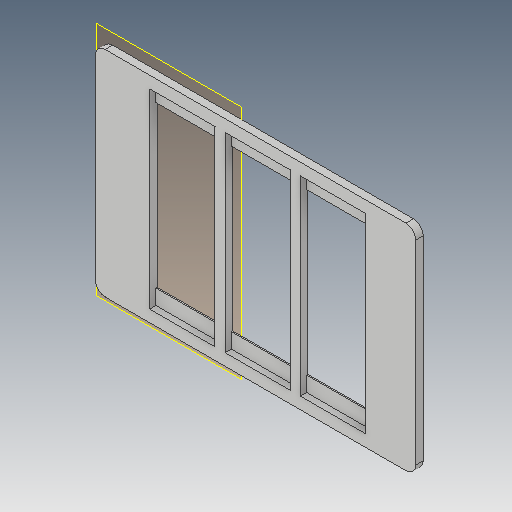
# Autodesk Inventor part: 30_MTP_wellplate_to_sample_adapter
Saved by Autodesk Inventor 2019.4 (Build 234330000, 330)
## iProperties
Created: 2021-05-14
Part Number: 30_MTP_wellplate_to_sample_adapter
Material: Generic
Document SubType Name: Modeling
Designer: diederichbenedict
Density: 1 g/cm^3
Appearance: Default
Author: diederichbenedict
Autodesk Inventor part; units mm, degrees
(part 1 of 2)
ref_plane "YZ Plane" through (0, 0, 0) normal (1, 0, 0) x (0, 1, 0)
ref_plane "XZ Plane" through (0, 0, 0) normal (0, 1, 0) x (-1, 0, 0)
ref_plane "XY Plane" through (0, 0, 0) normal (0, 0, 1) x (1, 0, 0)
ref_plane "Work Plane1" through (-0.8521, 0, -25.0767) normal (0, 0, 1) x (1, 0, 0)
sketch "Sketch1" plane through (-0.8521, 0, -25.0767) normal (0, 0, 1) x (1, 0, 0)
  line L0 (-59.9, 42.7) -> (-11.2, 42.7) projected
  arc A0 (-59.9, 42.7) -> (-63.8, 38.8) centre (-59.9, 38.8) ccw projected
  line L1 (-63.8, -38.8) -> (-63.8, 38.8) projected
  arc A1 (-63.8, -38.8) -> (-59.9, -42.7) centre (-59.9, -38.8) ccw projected
  line L2 (-11.2, -42.7) -> (-59.9, -42.7) projected
  line L3 (-11.2, -41.2) -> (-11.2, -42.7) projected
  line L4 (-55.7858, -41.2) -> (-11.2, -41.2) projected
  arc A2 (-56.5636, -40.8778) -> (-55.7858, -41.2) centre (-55.7858, -40.1) ccw projected
  line L5 (-61.9778, -35.4636) -> (-56.5636, -40.8778) projected
  arc A3 (-62.3, -34.6858) -> (-61.9778, -35.4636) centre (-61.2, -34.6858) ccw projected
  line L6 (-62.3, 34.6858) -> (-62.3, -34.6858) projected
  arc A4 (-61.9778, 35.4636) -> (-62.3, 34.6858) centre (-61.2, 34.6858) ccw projected
  line L7 (-56.5636, 40.8778) -> (-61.9778, 35.4636) projected
  arc A5 (-55.7858, 41.2) -> (-56.5636, 40.8778) centre (-55.7858, 40.1) ccw projected
  line L8 (-11.2, 41.2) -> (-55.7858, 41.2) projected
  line L9 (-11.2, 42.7) -> (-11.2, 41.2) projected
  line L10 (11.2, 42.7) -> (59.9, 42.7) projected
  line L11 (11.2, 41.2) -> (11.2, 42.7) projected
  line L12 (60.2, 41.2) -> (11.2, 41.2) projected
  arc A6 (62.3, 39.1) -> (60.2, 41.2) centre (60.2, 39.1) ccw projected
  line L13 (62.3, -39.1) -> (62.3, 39.1) projected
  arc A7 (60.2, -41.2) -> (62.3, -39.1) centre (60.2, -39.1) ccw projected
  line L14 (11.2, -41.2) -> (60.2, -41.2) projected
  line L15 (11.2, -42.7) -> (11.2, -41.2) projected
  line L16 (59.9, -42.7) -> (11.2, -42.7) projected
  arc A8 (59.9, -42.7) -> (63.8, -38.8) centre (59.9, -38.8) ccw projected
  line L17 (63.8, 38.8) -> (63.8, -38.8) projected
  arc A9 (63.8, 38.8) -> (59.9, 42.7) centre (59.9, 38.8) ccw projected
  line L18 (-11.2, 42.7) -> (11.2, 42.7)
  line L19 (-11.2, -42.7) -> (11.2, -42.7)
  point P0 (0.8521, 0)
  constraints: 4 end point, 1 horizontal, 1 parallel
extrude "Extrusion1" add sketch "Sketch1" along normal blind 3
sketch "Sketch2" plane through (-0.8521, 0, -22.0767) normal (0, 0, 1) x (1, 0, 0)
  line L0 (-61.4, -34.7272) -> (-61.4, 34.7272)
  arc A0 (-61.4, -34.7272) -> (-61.3707, -34.7979) centre (-61.3, -34.7272) ccw
  line L1 (-55.8979, -40.2707) -> (-61.3707, -34.7979)
  arc A1 (-55.8979, -40.2707) -> (-55.8272, -40.3) centre (-55.8272, -40.2) ccw
  line L2 (60.2, -40.3) -> (-55.8272, -40.3)
  arc A2 (60.2, -40.3) -> (61.4, -39.1) centre (60.2, -39.1) ccw
  line L3 (61.4, 39.1) -> (61.4, -39.1)
  arc A3 (61.4, 39.1) -> (60.2, 40.3) centre (60.2, 39.1) ccw
  line L4 (-55.8272, 40.3) -> (60.2, 40.3)
  arc A4 (-55.8272, 40.3) -> (-55.8979, 40.2707) centre (-55.8272, 40.2) ccw
  line L5 (-61.3707, 34.7979) -> (-55.8979, 40.2707)
  arc A5 (-61.3707, 34.7979) -> (-61.4, 34.7272) centre (-61.3, 34.7272) ccw
  spline S0 degree 3 poles (49.9248, 38.5524) (49.9706, 38.5524) (50.0527, 38.566) (50.1178, 38.6175) (50.1923, 38.7095) (50.2262, 38.788) (50.264, 38.8977) (50.2786, 38.9385) (50.2962, 38.9824) (50.3043, 39.0004) (50.3085, 39.0093) (50.3118, 39.0154) (50.3138, 39.0188) (50.3148, 39.0205) (50.3154, 39.0213) knots 0 0 0 0 0.208917 0.365604 0.365604 0.74824 0.74824 0.892103 0.946051 0.964034 0.982017 0.991009 0.995504 1 1 1 1
  spline S1 degree 3 poles (49.6421, 38.8514) (49.6421, 38.8062) (49.6542, 38.7253) (49.6991, 38.6574) (49.7455, 38.6109) (49.8073, 38.5666) (49.8825, 38.5524) (49.9248, 38.5524) knots 0 0 0 0 0.295249 0.516686 0.516686 0.723821 1 1 1 1
  spline S2 degree 3 poles (50.6998, 39.7369) (50.5423, 39.7369) (50.3824, 39.7163) (50.1145, 39.6094) (49.9987, 39.5409) (49.8226, 39.3665) (49.7538, 39.2676) (49.6682, 39.0616) (49.6421, 38.9566) (49.6421, 38.8514) knots 0 0 0 0 0.309207 0.309207 0.564439 0.564439 0.793646 0.793646 1 1 1 1
  spline S3 degree 3 poles (51.2464, 39.6371) (51.0757, 39.7115) (50.886, 39.7369) (50.6998, 39.7369) knots 0 0 0 0 1 1 1 1
  spline S4 degree 3 poles (51.7483, 38.8468) (51.7483, 38.9569) (51.7265, 39.0691) (51.6446, 39.273) (51.5842, 39.3684) (51.4343, 39.5265) (51.3443, 39.5914) (51.2464, 39.6371) knots 0 0 0 0 0.336501 0.336501 0.670162 0.670162 1 1 1 1
  spline S5 degree 3 poles (50.5143, 37.292) (50.5146, 37.2924) (50.5149, 37.2927) (50.5653, 37.3547) (50.632, 37.4188) (50.7687, 37.5437) (50.8504, 37.6122) (50.985, 37.7225) (51.13, 37.8422) (51.2754, 37.964) (51.4009, 38.0759) (51.4964, 38.1798) (51.576, 38.2978) (51.6548, 38.4286) (51.7244, 38.5813) (51.7483, 38.7514) (51.7483, 38.8468) knots 0 0 0 0 0.000671 0.000671 0.117108 0.136514 0.272358 0.272358 0.390523 0.548077 0.548077 0.63684 0.755191 0.755191 0.860109 1 1 1 1
  spline S6 degree 3 poles (50.4739, 37.2443) (50.4865, 37.2603) (50.4996, 37.2759) (50.5137, 37.2913) (50.514, 37.2916) (50.5143, 37.292) knots 0 0 0 0 0.977173 0.977173 1 1 1 1
  line L6 (51.426, 37.2443) -> (50.4739, 37.2443)
  spline S7 degree 3 poles (51.7995, 36.9546) (51.7995, 37.0015) (51.7819, 37.0846) (51.7254, 37.1482) (51.6221, 37.2283) (51.521, 37.2443) (51.426, 37.2443) knots 0 0 0 0 0.264865 0.463514 0.463514 1 1 1 1
  spline S8 degree 3 poles (51.4842, 36.6695) (51.5329, 36.6695) (51.6192, 36.6803) (51.6938, 36.7272) (51.7484, 36.7837) (51.7888, 36.8482) (51.7995, 36.923) (51.7995, 36.9546) knots 0 0 0 0 0.306499 0.536374 0.536374 0.801303 1 1 1 1
  line L7 (50.004, 36.6695) -> (51.4842, 36.6695)
  spline S9 degree 3 poles (49.6351, 36.9988) (49.6351, 36.9499) (49.6546, 36.8638) (49.7075, 36.794) (49.7632, 36.7383) (49.848, 36.6835) (49.948, 36.6695) (50.004, 36.6695) knots 0 0 0 0 0.266651 0.46664 0.46664 0.695223 1 1 1 1
  spline S10 degree 3 poles (49.8211, 37.4149) (49.8132, 37.4065) (49.8019, 37.3935) (49.7769, 37.3619) (49.7383, 37.3047) (49.7094, 37.2481) (49.6757, 37.1726) (49.6488, 37.1039) (49.6351, 37.0304) (49.6351, 36.9988) knots 0 0 0 0 0.074542 0.111813 0.260897 0.521795 0.521795 0.795055 1 1 1 1
  spline S11 degree 3 poles (50.6202, 38.1571) (50.5555, 38.1134) (50.4521, 38.0235) (50.3497, 37.9319) (50.1394, 37.7386) (49.9787, 37.5781) (49.8211, 37.4149) knots 0 0 0 0 0.214858 0.376351 0.376351 1 1 1 1
  spline S12 degree 3 poles (51.0967, 38.8351) (51.0967, 38.7587) (51.0761, 38.6824) (51.0056, 38.5283) (50.9498, 38.4518) (50.8073, 38.2986) (50.7155, 38.2242) (50.6202, 38.1571) knots 0 0 0 0 0.267675 0.267675 0.592009 0.592009 1 1 1 1
  spline S13 degree 3 poles (50.6882, 39.2297) (50.7597, 39.2297) (50.8316, 39.2135) (50.9555, 39.1474) (51.0068, 39.0985) (51.0792, 38.9784) (51.0967, 38.9062) (51.0967, 38.8351) knots 0 0 0 0 0.339544 0.339544 0.662755 0.662755 1 1 1 1
  spline S14 degree 3 poles (50.3154, 39.0213) (50.327, 39.039) (50.3522, 39.0735) (50.4027, 39.1277) (50.506, 39.206) (50.6141, 39.2297) (50.6882, 39.2297) knots 0 0 0 0 0.142857 0.285714 0.5 1 1 1 1
  spline S15 degree 3 poles (41.8364, 39.7748) (41.811, 39.7748) (41.7683, 39.7721) (41.7109, 39.7549) (41.6823, 39.7353) (41.6626, 39.7142) (41.6474, 39.696) (41.6219, 39.6634) (41.5791, 39.6066) (41.5442, 39.5585) (41.4471, 39.4233) (41.3629, 39.3308) (41.2056, 39.1936) (41.0994, 39.1226) (40.9771, 39.0575) (40.9199, 39.0295) (40.9008, 39.0204) (40.8912, 39.016) knots 0 0 0 0 0.061317 0.102194 0.143072 0.143072 0.171594 0.200115 0.242897 0.342722 0.342722 0.642421 0.642421 0.846752 0.948917 0.974459 1 1 1 1
  spline S16 degree 3 poles (42.1214, 39.4152) (42.1214, 39.506) (42.1029, 39.6005) (42.0257, 39.7002) (41.9644, 39.7561) (41.8824, 39.7748) (41.8364, 39.7748) knots 0 0 0 0 0.529945 0.529945 0.731397 1 1 1 1
  line L8 (42.1214, 37.1111) -> (42.1214, 39.4152)
  spline S17 degree 3 poles (41.7968, 36.6561) (41.8419, 36.6561) (41.9342, 36.6703) (42.0557, 36.7695) (42.1134, 36.9303) (42.1214, 37.051) (42.1214, 37.1111) knots 0 0 0 0 0.214286 0.428571 0.714286 1 1 1 1
  spline S18 degree 3 poles (41.4745, 37.032) (41.4745, 36.9337) (41.4957, 36.8286) (41.587, 36.7274) (41.6581, 36.6727) (41.747, 36.6561) (41.7968, 36.6561) knots 0 0 0 0 0.52997 0.52997 0.731411 1 1 1 1
  line L9 (41.4745, 38.763) -> (41.4745, 37.032)
  spline S19 degree 3 poles (40.8356, 38.4203) (40.8753, 38.4203) (40.953, 38.4406) (41.0976, 38.5077) (41.2717, 38.6159) (41.406, 38.7119) (41.4745, 38.763) knots 0 0 0 0 0.162539 0.325077 0.650155 1 1 1 1
  spline S20 degree 3 poles (40.5715, 38.6937) (40.5715, 38.6535) (40.5871, 38.583) (40.6296, 38.5249) (40.6782, 38.4745) (40.7359, 38.433) (40.806, 38.4203) (40.8356, 38.4203) knots 0 0 0 0 0.288261 0.504456 0.504456 0.787624 1 1 1 1
  spline S21 degree 3 poles (40.8912, 39.016) (40.8446, 38.994) (40.7636, 38.9541) (40.6859, 38.9082) (40.6306, 38.866) (40.5836, 38.8084) (40.5715, 38.7348) (40.5715, 38.6937) knots 0 0 0 0 0.317971 0.55645 0.55645 0.746543 1 1 1 1
  spline S22 degree 3 poles (32.6206, 39.7946) (32.4223, 39.7946) (32.2192, 39.7464) (31.8861, 39.5232) (31.7648, 39.3536) (31.6897, 39.1696) knots 0 0 0 0 0.499482 0.499482 1 1 1 1
  spline S23 degree 3 poles (33.555, 39.1791) (33.4987, 39.3021) (33.4239, 39.4196) (33.2403, 39.6048) (33.1316, 39.6769) (32.891, 39.7732) (32.7541, 39.7946) (32.6206, 39.7946) knots 0 0 0 0 0.343055 0.343055 0.661373 0.661373 1 1 1 1
  spline S24 degree 3 poles (33.7132, 38.2202) (33.7132, 38.3831) (33.6978, 38.7091) (33.6236, 39.0314) (33.555, 39.1791) knots 0 0 0 0 0.500073 1 1 1 1
  spline S25 degree 3 poles (33.5182, 37.1948) (33.5947, 37.3329) (33.6452, 37.4871) (33.7043, 37.833) (33.7132, 38.0272) (33.7132, 38.2202) knots 0 0 0 0 0.449932 0.449932 1 1 1 1
  spline S26 degree 3 poles (32.6369, 36.676) (32.8132, 36.676) (32.9919, 36.7208) (33.3013, 36.9028) (33.4283, 37.0393) (33.5182, 37.1948) knots 0 0 0 0 0.495402 0.495402 1 1 1 1
  spline S27 degree 3 poles (31.6779, 37.3597) (31.7561, 37.1627) (31.8857, 36.9828) (32.2271, 36.7393) (32.433, 36.676) (32.6369, 36.676) knots 0 0 0 0 0.509682 0.509682 1 1 1 1
  spline S28 degree 3 poles (31.5535, 38.1853) (31.5535, 38.0367) (31.562, 37.8877) (31.6017, 37.6111) (31.6319, 37.4822) (31.6779, 37.3597) knots 0 0 0 0 0.531664 0.531664 1 1 1 1
  spline S29 degree 3 poles (31.6897, 39.1696) (31.6366, 39.0323) (31.6061, 38.886) (31.5619, 38.5564) (31.5535, 38.3705) (31.5535, 38.1853) knots 0 0 0 0 0.442902 0.442902 1 1 1 1
  spline S30 degree 3 poles (12.4807, 38.9725) (12.4807, 38.8929) (12.5025, 38.731) (12.6264, 38.5139) (12.7575, 38.4103) (12.8305, 38.3667) knots 0 0 0 0 0.326804 0.653608 1 1 1 1
  spline S31 degree 3 poles (13.4594, 39.7929) (13.2813, 39.7929) (13.1007, 39.7611) (12.8035, 39.6109) (12.6805, 39.5087) (12.5235, 39.2558) (12.4807, 39.114) (12.4807, 38.9725) knots 0 0 0 0 0.376521 0.376521 0.700973 0.700973 1 1 1 1
  spline S32 degree 3 poles (14.4682, 38.9679) (14.4682, 39.0742) (14.4476, 39.1826) (14.3635, 39.3811) (14.2955, 39.4716) (14.1233, 39.6272) (14.0117, 39.6869) (13.757, 39.7757) (13.6062, 39.7929) (13.4594, 39.7929) knots 0 0 0 0 0.21947 0.21947 0.444496 0.444496 0.697041 0.697041 1 1 1 1
  spline S33 degree 3 poles (14.1258, 38.3673) (14.2175, 38.4243) (14.2996, 38.4973) (14.4323, 38.7002) (14.4682, 38.835) (14.4682, 38.9679) knots 0 0 0 0 0.446505 0.446505 1 1 1 1
  spline S34 degree 3 poles (14.5753, 37.625) (14.5753, 37.7377) (14.5567, 37.8531) (14.4745, 38.0579) (14.4111, 38.1502) (14.272, 38.2821) (14.2011, 38.3293) (14.1258, 38.3673) knots 0 0 0 0 0.370643 0.370643 0.72504 0.72504 1 1 1 1
  spline S35 degree 3 poles (13.4826, 36.6743) (13.6825, 36.6743) (13.8855, 36.7075) (14.2207, 36.8718) (14.3578, 36.989) (14.5327, 37.2854) (14.5753, 37.4563) (14.5753, 37.625) knots 0 0 0 0 0.369586 0.369586 0.688081 0.688081 1 1 1 1
  spline S36 degree 3 poles (12.383, 37.6203) (12.383, 37.4518) (12.4245, 37.2827) (12.5988, 36.9876) (12.7355, 36.8717) (13.0732, 36.7061) (13.2805, 36.6743) (13.4826, 36.6743) knots 0 0 0 0 0.310931 0.310931 0.627014 0.627014 1 1 1 1
  spline S37 degree 3 poles (12.8305, 38.3667) (12.7745, 38.3387) (12.6372, 38.2544) (12.4308, 38.017) (12.383, 37.7663) (12.383, 37.6203) knots 0 0 0 0 0.203868 0.522321 1 1 1 1
  spline S38 degree 3 poles (-4.416, 39.3012) (-4.3747, 39.3012) (-4.301, 39.2902) (-4.2367, 39.2557) (-4.186, 39.219) (-4.1325, 39.1694) (-4.0961, 39.1049) (-4.0813, 39.0665) knots 0 0 0 0 0.285623 0.49984 0.49984 0.715083 1 1 1 1
  spline S39 degree 3 poles (-4.7635, 39.0948) (-4.7215, 39.1558) (-4.6666, 39.2087) (-4.5459, 39.2797) (-4.4812, 39.3012) (-4.416, 39.3012) knots 0 0 0 0 0.531786 0.531786 1 1 1 1
  spline S40 degree 3 poles (-4.92, 38.4993) (-4.9117, 38.5979) (-4.892, 38.75) (-4.8395, 38.9502) (-4.7943, 39.0503) (-4.7635, 39.0948) knots 0 0 0 0 0.476274 0.738137 1 1 1 1
  spline S41 degree 3 poles (-4.3206, 38.7333) (-4.4514, 38.7333) (-4.5851, 38.7076) (-4.7825, 38.6117) (-4.8549, 38.5596) (-4.92, 38.4993) knots 0 0 0 0 0.59802 0.59802 1 1 1 1
  spline S42 degree 3 poles (-3.3792, 37.7221) (-3.3792, 37.8552) (-3.4023, 37.9889) (-3.4932, 38.2345) (-3.5602, 38.3479) (-3.7313, 38.5337) (-3.8346, 38.6084) (-4.0642, 38.7091) (-4.1937, 38.7333) (-4.3206, 38.7333) knots 0 0 0 0 0.260333 0.260333 0.510573 0.510573 0.752032 0.752032 1 1 1 1
  spline S43 degree 3 poles (-4.4462, 36.6666) (-4.2555, 36.6666) (-4.0635, 36.7094) (-3.7369, 36.8923) (-3.6035, 37.0252) (-3.4234, 37.3481) (-3.3792, 37.5364) (-3.3792, 37.7221) knots 0 0 0 0 0.3423 0.3423 0.666781 0.666781 1 1 1 1
  spline S44 degree 3 poles (-5.5855, 38.1596) (-5.5855, 37.8852) (-5.5545, 37.6055) (-5.3701, 37.1493) (-5.2399, 36.9631) (-4.8794, 36.7194) (-4.6602, 36.6666) (-4.4462, 36.6666) knots 0 0 0 0 0.389095 0.389095 0.69658 0.69658 1 1 1 1
  spline S45 degree 3 poles (-4.3997, 39.7852) (-4.5703, 39.7852) (-4.7435, 39.7541) (-5.0446, 39.6095) (-5.1736, 39.4986) (-5.3853, 39.2153) (-5.4583, 39.0349) (-5.5642, 38.6271) (-5.5855, 38.3912) (-5.5855, 38.1596) knots 0 0 0 0 0.226159 0.226159 0.442737 0.442737 0.693049 0.693049 1 1 1 1
  spline S46 degree 3 poles (-3.5002, 39.0999) (-3.5002, 39.2117) (-3.545, 39.3198) (-3.6845, 39.5298) (-3.7983, 39.6168) (-4.0687, 39.7544) (-4.2361, 39.7852) (-4.3997, 39.7852) knots 0 0 0 0 0.27049 0.27049 0.604259 0.604259 1 1 1 1
  spline S47 degree 3 poles (-3.7713, 38.8334) (-3.7301, 38.8334) (-3.6574, 38.848) (-3.598, 38.8929) (-3.55, 38.9436) (-3.5116, 39.0019) (-3.5002, 39.0708) (-3.5002, 39.0999) knots 0 0 0 0 0.294434 0.515259 0.515259 0.792254 1 1 1 1
  spline S48 degree 3 poles (-4.0813, 39.0665) (-4.0581, 38.999) (-4.016, 38.9369) (-3.9033, 38.8564) (-3.8373, 38.8334) (-3.7713, 38.8334) knots 0 0 0 0 0.519251 0.519251 1 1 1 1
  spline S49 degree 3 poles (-31.6269, 37.164) (-31.682, 37.164) (-31.7622, 37.1743) (-31.8622, 37.2228) (-31.9049, 37.2596) (-31.9544, 37.3158) (-32.0047, 37.3874) (-32.0761, 37.5211) (-32.1179, 37.6217) (-32.1407, 37.6824) knots 0 0 0 0 0.210336 0.30048 0.420672 0.420672 0.586503 0.752334 1 1 1 1
  spline S50 degree 3 poles (-31.1695, 37.6377) (-31.1695, 37.5498) (-31.1906, 37.4601) (-31.2803, 37.3166) (-31.3386, 37.2578) (-31.4764, 37.184) (-31.5518, 37.164) (-31.6269, 37.164) knots 0 0 0 0 0.362038 0.362038 0.690804 0.690804 1 1 1 1
  spline S51 degree 3 poles (-31.606, 38.0927) (-31.5475, 38.0927) (-31.4631, 38.0827) (-31.3551, 38.0351) (-31.3079, 37.9982) (-31.2487, 37.9369) (-31.1845, 37.8303) (-31.1695, 37.7067) (-31.1695, 37.6377) knots 0 0 0 0 0.245945 0.35135 0.49189 0.49189 0.709651 1 1 1 1
  spline S52 degree 3 poles (-31.8387, 38.0764) (-31.8279, 38.0764) (-31.8064, 38.0777) (-31.7687, 38.0807) (-31.7418, 38.0832) (-31.703, 38.087) (-31.663, 38.0905) (-31.6231, 38.0927) (-31.606, 38.0927) knots 0 0 0 0 0.138756 0.277512 0.485646 0.485646 0.779562 1 1 1 1
  spline S53 degree 3 poles (-32.1214, 38.3359) (-32.1214, 38.2958) (-32.1096, 38.2248) (-32.067, 38.166) (-32.0216, 38.1241) (-31.9561, 38.0858) (-31.8809, 38.0764) (-31.8387, 38.0764) knots 0 0 0 0 0.278638 0.487616 0.487616 0.707209 1 1 1 1
  spline S54 degree 3 poles (-31.7829, 38.6) (-31.87, 38.6) (-31.9632, 38.5851) (-32.0555, 38.5092) (-32.1048, 38.4523) (-32.1214, 38.3777) (-32.1214, 38.3359) knots 0 0 0 0 0.543347 0.543347 0.739056 1 1 1 1
  line L10 (-31.7014, 38.6) -> (-31.7829, 38.6)
  spline S55 degree 3 poles (-31.2976, 38.9713) (-31.2976, 38.9202) (-31.3073, 38.8456) (-31.3545, 38.7538) (-31.39, 38.7155) (-31.4587, 38.66) (-31.5526, 38.6117) (-31.6573, 38.6) (-31.7014, 38.6) knots 0 0 0 0 0.24907 0.355815 0.498141 0.498141 0.784917 1 1 1 1
  spline S56 degree 3 poles (-31.6432, 39.2983) (-31.5904, 39.2983) (-31.4968, 39.2848) (-31.4181, 39.2306) (-31.3573, 39.1671) (-31.3098, 39.0937) (-31.2976, 39.0075) (-31.2976, 38.9713) knots 0 0 0 0 0.298234 0.521909 0.521909 0.795104 1 1 1 1
  spline S57 degree 3 poles (-32.0885, 38.8906) (-32.064, 38.9463) (-32.0384, 39.0019) (-31.9897, 39.1046) (-31.9641, 39.1512) (-31.9038, 39.227) (-31.8655, 39.2515) (-31.7683, 39.2923) (-31.7047, 39.2983) (-31.6432, 39.2983) knots 0 0 0 0 0.27828 0.27828 0.519339 0.519339 0.719009 0.719009 1 1 1 1
  spline S58 degree 3 poles (-32.3275, 38.7723) (-32.2788, 38.7723) (-32.2294, 38.7801) (-32.1644, 38.809) (-32.1336, 38.8278) (-32.1057, 38.8594) (-32.094, 38.8789) (-32.0898, 38.8876) (-32.0885, 38.8906) knots 0 0 0 0 0.519817 0.519817 0.759908 0.897104 0.965701 1 1 1 1
  spline S59 degree 3 poles (-32.5916, 39.0597) (-32.5916, 39.016) (-32.5782, 38.9387) (-32.5325, 38.8744) (-32.481, 38.8247) (-32.4244, 38.7851) (-32.3563, 38.7723) (-32.3275, 38.7723) knots 0 0 0 0 0.303995 0.531992 0.531992 0.799425 1 1 1 1
  spline S60 degree 3 poles (-31.5874, 39.7823) (-31.7291, 39.7823) (-31.8719, 39.7633) (-32.122, 39.6767) (-32.2327, 39.62) (-32.4046, 39.4727) (-32.4739, 39.3951) (-32.5635, 39.229) (-32.5916, 39.145) (-32.5916, 39.0597) knots 0 0 0 0 0.314119 0.314119 0.584504 0.584504 0.810964 0.810964 1 1 1 1
  spline S61 degree 3 poles (-30.6599, 39.0062) (-30.6599, 39.1109) (-30.6813, 39.2176) (-30.7688, 39.4094) (-30.8364, 39.4951) (-31.0042, 39.6365) (-31.1068, 39.6907) (-31.3338, 39.7658) (-31.462, 39.7823) (-31.5874, 39.7823) knots 0 0 0 0 0.233642 0.233642 0.468764 0.468764 0.720482 0.720482 1 1 1 1
  spline S62 degree 3 poles (-30.9639, 38.3907) (-30.8842, 38.4628) (-30.812, 38.5437) (-30.6882, 38.7458) (-30.6599, 38.8776) (-30.6599, 39.0062) knots 0 0 0 0 0.454637 0.454637 1 1 1 1
  spline S63 degree 3 poles (-30.518, 37.6633) (-30.518, 37.7666) (-30.5368, 37.8722) (-30.616, 38.0625) (-30.6765, 38.1501) (-30.8126, 38.2877) (-30.8861, 38.3432) (-30.9639, 38.3906) knots 0 0 0 0 0.348008 0.348008 0.69452 0.69452 1 1 1 1
  spline S64 degree 3 poles (-31.6316, 36.6684) (-31.4788, 36.6684) (-31.3224, 36.6924) (-31.0492, 36.7974) (-30.9256, 36.8715) (-30.7273, 37.057) (-30.6472, 37.1676) (-30.545, 37.406) (-30.518, 37.5357) (-30.518, 37.6633) knots 0 0 0 0 0.277081 0.277081 0.529944 0.529944 0.768625 0.768625 1 1 1 1
  spline S65 degree 3 poles (-32.6777, 37.5213) (-32.6777, 37.484) (-32.6625, 37.3971) (-32.6309, 37.3158) (-32.563, 37.1649) (-32.4937, 37.0701) (-32.3205, 36.8889) (-32.2053, 36.8142) (-31.9424, 36.6956) (-31.7852, 36.6684) (-31.6316, 36.6684) knots 0 0 0 0 0.076031 0.177405 0.177405 0.41271 0.41271 0.686557 0.686557 1 1 1 1
  spline S66 degree 3 poles (-32.3647, 37.8296) (-32.4108, 37.8296) (-32.4922, 37.815) (-32.561, 37.7689) (-32.6207, 37.7128) (-32.6669, 37.6406) (-32.6777, 37.5567) (-32.6777, 37.5213) knots 0 0 0 0 0.282671 0.494675 0.494675 0.783432 1 1 1 1
  spline S67 degree 3 poles (-32.1407, 37.6824) (-32.1493, 37.7078) (-32.1751, 37.7493) (-32.2126, 37.7786) (-32.2705, 37.8147) (-32.3175, 37.8296) (-32.3647, 37.8296) knots 0 0 0 0 0.284325 0.500225 0.500225 1 1 1 1
  spline S68 degree 3 poles (-49.2727, 39.7969) (-49.3066, 39.7969) (-49.3667, 39.7924) (-49.421, 39.7636) (-49.4546, 39.7277) (-49.4801, 39.6951) (-49.5301, 39.6289) (-49.5648, 39.5806) (-49.662, 39.4454) (-49.7461, 39.353) (-49.9035, 39.2158) (-50.0274, 39.1329) (-50.1604, 39.065) (-50.2179, 39.0381) knots 0 0 0 0 0.081756 0.143072 0.143072 0.200115 0.242897 0.342722 0.342722 0.642421 0.642421 0.846752 1 1 1 1
  spline S69 degree 3 poles (-48.9876, 39.4374) (-48.9876, 39.5281) (-49.0061, 39.6227) (-49.0834, 39.7224) (-49.1446, 39.7782) (-49.2267, 39.7969) (-49.2727, 39.7969) knots 0 0 0 0 0.529945 0.529945 0.731397 1 1 1 1
  line L11 (-48.9876, 37.1333) -> (-48.9876, 39.4374)
  spline S70 degree 3 poles (-49.3123, 36.6783) (-49.2521, 36.6783) (-49.1271, 36.7073) (-49.0255, 36.85) (-48.993, 36.997) (-48.9876, 37.0882) (-48.9876, 37.1333) knots 0 0 0 0 0.285714 0.571429 0.785714 1 1 1 1
  spline S71 degree 3 poles (-49.6346, 37.0541) (-49.6346, 36.9558) (-49.6133, 36.8508) (-49.5137, 36.7403) (-49.4384, 36.6901) (-49.3496, 36.6783) (-49.3123, 36.6783) knots 0 0 0 0 0.52997 0.52997 0.798558 1 1 1 1
  line L12 (-49.6346, 38.7852) -> (-49.6346, 37.0541)
  spline S72 degree 3 poles (-50.2735, 38.4425) (-50.2338, 38.4425) (-50.1561, 38.4627) (-50.0114, 38.5299) (-49.8374, 38.638) (-49.7031, 38.734) (-49.6346, 38.7852) knots 0 0 0 0 0.162539 0.325077 0.650155 1 1 1 1
  spline S73 degree 3 poles (-50.5376, 38.7159) (-50.5376, 38.6757) (-50.522, 38.6052) (-50.4794, 38.547) (-50.4308, 38.4967) (-50.3732, 38.4551) (-50.3031, 38.4425) (-50.2735, 38.4425) knots 0 0 0 0 0.288261 0.504456 0.504456 0.787624 1 1 1 1
  spline S74 degree 3 poles (-50.2179, 39.0381) (-50.2644, 39.0162) (-50.3454, 38.9762) (-50.4232, 38.9304) (-50.4784, 38.8882) (-50.5255, 38.8305) (-50.5376, 38.7569) (-50.5376, 38.7159) knots 0 0 0 0 0.317971 0.55645 0.55645 0.746543 1 1 1 1
  spline S75 degree 3 poles (-57.034, 20.7963) (-56.895, 20.7963) (-56.7555, 20.8016) (-56.5077, 20.8347) (-56.3977, 20.8603) (-56.2951, 20.9027) knots 0 0 0 0 0.555853 0.555853 1 1 1 1
  line L13 (-57.9347, 20.7963) -> (-57.034, 20.7963)
  spline S76 degree 3 poles (-58.3455, 21.2117) (-58.3455, 21.1001) (-58.3254, 20.9798) (-58.1695, 20.8175) (-58.047, 20.7963) (-57.9347, 20.7963) knots 0 0 0 0 0.498316 0.498316 1 1 1 1
  line L14 (-58.3455, 23.4297) -> (-58.3455, 21.2117)
  spline S77 degree 3 poles (-57.9347, 23.8451) (-58.0461, 23.8451) (-58.1667, 23.8246) (-58.326, 23.6654) (-58.3455, 23.5424) (-58.3455, 23.4297) knots 0 0 0 0 0.496968 0.496968 1 1 1 1
  line L15 (-56.9782, 23.8451) -> (-57.9347, 23.8451)
  spline S78 degree 3 poles (-56.31, 23.7122) (-56.3997, 23.7664) (-56.5024, 23.8017) (-56.7285, 23.8391) (-56.8537, 23.8451) (-56.9782, 23.8451) knots 0 0 0 0 0.457185 0.457185 1 1 1 1
  spline S79 degree 3 poles (-55.9367, 23.055) (-55.9367, 23.1439) (-55.9511, 23.2338) (-56.0114, 23.3996) (-56.0562, 23.4764) (-56.1684, 23.6097) (-56.2359, 23.6677) (-56.31, 23.7122) knots 0 0 0 0 0.338894 0.338894 0.67071 0.67071 1 1 1 1
  spline S80 degree 3 poles (-56.306, 22.4163) (-56.1931, 22.4847) (-55.9956, 22.6635) (-55.9367, 22.9284) (-55.9367, 23.055) knots 0 0 0 0 0.507785 1 1 1 1
  spline S81 degree 3 poles (-55.7971, 21.6865) (-55.7971, 21.7875) (-55.8265, 21.9935) (-56.0107, 22.2624) (-56.2001, 22.3725) (-56.306, 22.4163) knots 0 0 0 0 0.320193 0.640385 1 1 1 1
  spline S82 degree 3 poles (-56.2951, 20.9027) (-56.148, 20.9683) (-56.0195, 21.0781) (-55.8421, 21.3548) (-55.797, 21.5217) (-55.7971, 21.6865) knots 0 0 0 0 0.494375 0.494375 1 1 1 1
  spline S83 degree 3 poles (-57.1318, 2.7963) (-57.0075, 2.7963) (-56.8816, 2.8031) (-56.6494, 2.8396) (-56.5427, 2.8705) (-56.3421, 2.9633) (-56.2501, 3.0251) (-56.1694, 3.0979) knots 0 0 0 0 0.362045 0.362045 0.683397 0.683397 1 1 1 1
  line L16 (-57.9091, 2.7963) -> (-57.1318, 2.7963)
  spline S84 degree 3 poles (-58.3385, 3.2675) (-58.3385, 3.1844) (-58.3339, 3.1003) (-58.2995, 2.9799) (-58.2647, 2.9142) (-58.207, 2.868) (-58.1455, 2.8317) (-58.0564, 2.8023) (-57.9622, 2.7963) (-57.9091, 2.7963) knots 0 0 0 0 0.334772 0.334772 0.501276 0.626154 0.626154 0.786374 1 1 1 1
  line L17 (-58.3385, 5.4297) -> (-58.3385, 3.2675)
  spline S85 degree 3 poles (-57.9231, 5.8451) (-58.0357, 5.8451) (-58.1564, 5.8257) (-58.319, 5.6633) (-58.3385, 5.5421) (-58.3385, 5.4297) knots 0 0 0 0 0.500349 0.500349 1 1 1 1
  line L18 (-57.1434, 5.8451) -> (-57.9231, 5.8451)
  spline S86 degree 3 poles (-56.196, 5.5652) (-56.3142, 5.6693) (-56.4582, 5.7485) (-56.7838, 5.832) (-56.9648, 5.8451) (-57.1434, 5.8451) knots 0 0 0 0 0.46869 0.46869 1 1 1 1
  spline S87 degree 3 poles (-55.7179, 4.3288) (-55.7179, 4.5559) (-55.7688, 5.0191) (-56.0234, 5.4178) (-56.196, 5.5652) knots 0 0 0 0 0.500147 1 1 1 1
  spline S88 degree 3 poles (-56.1694, 3.0979) (-56.0677, 3.1917) (-55.9807, 3.3025) (-55.8435, 3.5536) (-55.7959, 3.6918) (-55.7311, 3.9963) (-55.7179, 4.164) (-55.7179, 4.3288) knots 0 0 0 0 0.308658 0.308658 0.632164 0.632164 1 1 1 1
  line L19 (-57.659, -14.8395) -> (-57.659, -13.9167)
  spline S89 degree 3 poles (-58.0069, -15.2549) (-57.9537, -15.2549) (-57.8594, -15.2364) (-57.7835, -15.1786) (-57.7131, -15.1034) (-57.6671, -14.9981) (-57.659, -14.8868) (-57.659, -14.8395) knots 0 0 0 0 0.261511 0.457644 0.457644 0.767562 1 1 1 1
  spline S90 degree 3 poles (-58.3548, -14.8419) (-58.3548, -14.9507) (-58.3319, -15.0677) (-58.2305, -15.1775) (-58.1548, -15.2361) (-58.0601, -15.2549) (-58.0069, -15.2549) knots 0 0 0 0 0.538985 0.538985 0.736563 1 1 1 1
  line L20 (-58.3548, -12.5703) -> (-58.3548, -14.8419)
  spline S91 degree 3 poles (-57.9394, -12.1549) (-58.017, -12.1549) (-58.0966, -12.1644) (-58.2031, -12.2131) (-58.2609, -12.2542) (-58.2989, -12.3126) (-58.3454, -12.4113) (-58.3548, -12.4918) (-58.3548, -12.5703) knots 0 0 0 0 0.345203 0.345203 0.519861 0.650854 0.650854 1 1 1 1
  line L21 (-56.5313, -12.1549) -> (-57.9394, -12.1549)
  spline S92 degree 3 poles (-56.1997, -12.4353) (-56.1997, -12.3919) (-56.214, -12.315) (-56.2618, -12.2524) (-56.3138, -12.2056) (-56.393, -12.1638) (-56.4816, -12.1549) (-56.5313, -12.1549) knots 0 0 0 0 0.266602 0.466553 0.466553 0.695173 1 1 1 1
  spline S93 degree 3 poles (-56.5313, -12.7158) (-56.4444, -12.7158) (-56.351, -12.6985) (-56.2536, -12.6109) (-56.21, -12.5452) (-56.1997, -12.4679) (-56.1997, -12.4353) knots 0 0 0 0 0.533679 0.533679 0.800148 1 1 1 1
  line L22 (-57.659, -12.7158) -> (-56.5313, -12.7158)
  line L23 (-57.659, -13.3698) -> (-57.659, -12.7158)
  line L24 (-56.7245, -13.3698) -> (-57.659, -13.3698)
  spline S94 degree 3 poles (-56.4045, -13.6433) (-56.4045, -13.6011) (-56.4187, -13.5266) (-56.4649, -13.4659) (-56.5149, -13.4203) (-56.5908, -13.3789) (-56.6764, -13.3698) (-56.7245, -13.3698) knots 0 0 0 0 0.267155 0.467521 0.467521 0.695726 1 1 1 1
  spline S95 degree 3 poles (-56.7245, -13.9167) (-56.6408, -13.9167) (-56.5512, -13.8995) (-56.4648, -13.8221) (-56.4184, -13.7613) (-56.4045, -13.6857) (-56.4045, -13.6433) knots 0 0 0 0 0.529874 0.529874 0.731356 1 1 1 1
  line L25 (-57.659, -13.9167) -> (-56.7245, -13.9167)
  line L26 (-56.451, -30.5168) -> (-56.451, -31.3116)
  spline S96 degree 3 poles (-56.1054, -30.1037) (-56.1589, -30.1037) (-56.2534, -30.1218) (-56.3299, -30.1812) (-56.3878, -30.2457) (-56.4398, -30.3444) (-56.451, -30.4548) (-56.451, -30.5168) knots 0 0 0 0 0.26477 0.463347 0.463347 0.693341 1 1 1 1
  spline S97 degree 3 poles (-55.7552, -30.5168) (-55.7552, -30.4074) (-55.7774, -30.2894) (-55.8891, -30.17) (-55.9701, -30.1167) (-56.0653, -30.1037) (-56.1054, -30.1037) knots 0 0 0 0 0.539039 0.539039 0.802445 1 1 1 1
  line L27 (-55.7552, -32.8395) -> (-55.7552, -30.5168)
  spline S98 degree 3 poles (-56.1054, -33.2549) (-56.0516, -33.2549) (-55.9563, -33.2364) (-55.8796, -33.1777) (-55.8203, -33.1135) (-55.7665, -33.0141) (-55.7552, -32.9023) (-55.7552, -32.8395) knots 0 0 0 0 0.263761 0.461581 0.461581 0.692332 1 1 1 1
  spline S99 degree 3 poles (-56.451, -32.8395) (-56.451, -32.9478) (-56.43, -33.0639) (-56.3227, -33.1867) (-56.2418, -33.242) (-56.1458, -33.2549) (-56.1054, -33.2549) knots 0 0 0 0 0.534609 0.534609 0.800547 1 1 1 1
  line L28 (-56.451, -31.8981) -> (-56.451, -32.8395)
  line L29 (-57.6427, -31.8981) -> (-56.451, -31.8981)
  line L30 (-57.6427, -32.8395) -> (-57.6427, -31.8981)
  spline S100 degree 3 poles (-57.9929, -33.2549) (-57.9391, -33.2549) (-57.8438, -33.2364) (-57.7671, -33.1777) (-57.7078, -33.1135) (-57.6541, -33.0141) (-57.6427, -32.9023) (-57.6427, -32.8395) knots 0 0 0 0 0.263761 0.461581 0.461581 0.692332 1 1 1 1
  spline S101 degree 3 poles (-58.3385, -32.8395) (-58.3385, -32.9478) (-58.3175, -33.0639) (-58.2102, -33.1867) (-58.1294, -33.242) (-58.0333, -33.2549) (-57.9929, -33.2549) knots 0 0 0 0 0.534609 0.534609 0.800547 1 1 1 1
  line L31 (-58.3385, -30.5168) -> (-58.3385, -32.8395)
  spline S102 degree 3 poles (-57.9929, -30.1037) (-58.047, -30.1037) (-58.1428, -30.121) (-58.2203, -30.181) (-58.2775, -30.2465) (-58.3278, -30.3453) (-58.3385, -30.4551) (-58.3385, -30.5168) knots 0 0 0 0 0.267096 0.467418 0.467418 0.695668 1 1 1 1
  spline S103 degree 3 poles (-57.6427, -30.5168) (-57.6427, -30.4074) (-57.6649, -30.2894) (-57.7766, -30.17) (-57.8576, -30.1167) (-57.9528, -30.1037) (-57.9929, -30.1037) knots 0 0 0 0 0.539039 0.539039 0.802445 1 1 1 1
  line L32 (-57.6427, -31.3116) -> (-57.6427, -30.5168)
  line L33 (-56.451, -31.3116) -> (-57.6427, -31.3116)
  arc A6 (-54.2, -35) -> (-53, -36.2) centre (-53, -35) ccw
  line L34 (-54.2, 35) -> (-54.2, -35)
  arc A7 (-53, 36.2) -> (-54.2, 35) centre (-53, 35) ccw
  line L35 (53, 36.2) -> (-53, 36.2)
  arc A8 (54.2, 35) -> (53, 36.2) centre (53, 35) ccw
  line L36 (54.2, -35) -> (54.2, 35)
  arc A9 (53, -36.2) -> (54.2, -35) centre (53, -35) ccw
  line L37 (-53, -36.2) -> (53, -36.2)
  line L38 (-56.6104, -23.1029) -> (-56.1973, -23.1029)
  spline S104 degree 3 poles (-56.9979, -22.8318) (-56.9979, -22.8797) (-56.9818, -22.9657) (-56.9195, -23.0276) (-56.853, -23.0667) (-56.7616, -23.0967) (-56.6648, -23.1029) (-56.6104, -23.1029) knots 0 0 0 0 0.267771 0.468599 0.468599 0.696342 1 1 1 1
  spline S105 degree 3 poles (-56.6826, -22.556) (-56.7176, -22.556) (-56.7996, -22.5638) (-56.8755, -22.6014) (-56.9421, -22.6615) (-56.9863, -22.7243) (-56.9979, -22.7999) (-56.9979, -22.8318) knots 0 0 0 0 0.224508 0.523853 0.523853 0.795937 1 1 1 1
  line L39 (-56.0053, -22.556) -> (-56.6826, -22.556)
  spline S106 degree 3 poles (-55.5503, -22.9551) (-55.5503, -22.9039) (-55.557, -22.8136) (-55.5908, -22.7285) (-55.636, -22.6645) (-55.6866, -22.6146) (-55.7522, -22.5871) (-55.854, -22.561) (-55.9301, -22.556) (-56.0053, -22.556) knots 0 0 0 0 0.2188 0.3829 0.3829 0.552067 0.678942 0.678942 1 1 1 1
  line L40 (-55.5503, -23.5207) -> (-55.5503, -22.9551)
  spline S107 degree 3 poles (-55.8324, -23.9719) (-55.7746, -23.9401) (-55.7187, -23.9037) (-55.6274, -23.8196) (-55.5929, -23.7703) (-55.5546, -23.6533) (-55.5503, -23.5861) (-55.5503, -23.5207) knots 0 0 0 0 0.348817 0.348817 0.654069 0.654069 1 1 1 1
  spline S108 degree 3 poles (-56.9107, -24.2549) (-56.725, -24.2549) (-56.5371, -24.2351) (-56.175, -24.1378) (-55.999, -24.0617) (-55.8324, -23.9719) knots 0 0 0 0 0.495343 0.495343 1 1 1 1
  spline S109 degree 3 poles (-58.4642, -22.6782) (-58.4642, -22.8996) (-58.4326, -23.1231) (-58.286, -23.5164) (-58.1801, -23.6911) (-57.9036, -23.9709) (-57.7308, -24.0782) (-57.3457, -24.2226) (-57.1256, -24.2549) (-56.9107, -24.2549) knots 0 0 0 0 0.26691 0.26691 0.504896 0.504896 0.740854 0.740854 1 1 1 1
  spline S110 degree 3 poles (-56.8781, -21.1037) (-57.1032, -21.1037) (-57.3307, -21.1344) (-57.7293, -21.2819) (-57.9051, -21.3886) (-58.1859, -21.6694) (-58.2919, -21.846) (-58.4322, -22.2382) (-58.4642, -22.4606) (-58.4642, -22.6782) knots 0 0 0 0 0.268167 0.268167 0.504846 0.504846 0.740886 0.740886 1 1 1 1
  spline S111 degree 3 poles (-55.6411, -21.9288) (-55.6411, -21.8365) (-55.6755, -21.7471) (-55.7749, -21.5612) (-55.8556, -21.4715) (-56.0592, -21.2994) (-56.1952, -21.2337) (-56.5079, -21.1258) (-56.6955, -21.1037) (-56.8781, -21.1037) knots 0 0 0 0 0.170978 0.170978 0.389439 0.389439 0.661596 0.661596 1 1 1 1
  spline S112 degree 3 poles (-55.9751, -22.2511) (-55.926, -22.2511) (-55.8397, -22.234) (-55.7674, -22.1837) (-55.7049, -22.1246) (-55.6547, -22.0522) (-55.6411, -21.9653) (-55.6411, -21.9288) knots 0 0 0 0 0.28653 0.501427 0.501427 0.786326 1 1 1 1
  spline S113 degree 3 poles (-56.2395, -22.1158) (-56.2389, -22.1165) (-56.2384, -22.1171) (-56.2063, -22.1581) (-56.1658, -22.192) (-56.0752, -22.2382) (-56.025, -22.2511) (-55.9751, -22.2511) knots 0 0 0 0 0.008527 0.008527 0.510352 0.510352 1 1 1 1
  spline S114 degree 3 poles (-56.9223, -21.6646) (-56.817, -21.6646) (-56.7074, -21.6756) (-56.5409, -21.7536) (-56.4739, -21.7975) (-56.3535, -21.9362) (-56.2964, -22.0249) (-56.2404, -22.1143) (-56.2399, -22.115) (-56.2395, -22.1158) knots 0 0 0 0 0.364357 0.364357 0.634905 0.634905 0.996992 0.996992 1 1 1 1
  spline S115 degree 3 poles (-57.759, -22.6642) (-57.759, -22.5217) (-57.7422, -22.3781) (-57.6639, -22.127) (-57.6099, -22.0167) (-57.4619, -21.8418) (-57.3719, -21.7748) (-57.1631, -21.6838) (-57.0412, -21.6646) (-56.9223, -21.6646) knots 0 0 0 0 0.291269 0.291269 0.535594 0.535594 0.757024 0.757024 1 1 1 1
  spline S116 degree 3 poles (-56.906, -23.6918) (-57.0226, -23.6918) (-57.2587, -23.6598) (-57.4565, -23.5189) (-57.7084, -23.224) (-57.759, -22.9344) (-57.759, -22.6642) knots 0 0 0 0 0.231589 0.463179 0.463179 1 1 1 1
  spline S117 degree 3 poles (-56.1973, -23.5022) (-56.3039, -23.5577) (-56.4155, -23.6048) (-56.6516, -23.6754) (-56.7796, -23.6918) (-56.906, -23.6918) knots 0 0 0 0 0.487157 0.487157 1 1 1 1
  line L41 (-56.1973, -23.1029) -> (-56.1973, -23.5022)
  line L42 (-56.3032, -5.6289) -> (-57.645, -5.6289)
  spline S118 degree 3 poles (-55.9693, -5.9187) (-55.9693, -5.8739) (-55.9834, -5.7949) (-56.0317, -5.73) (-56.0842, -5.6818) (-56.1635, -5.6384) (-56.253, -5.6289) (-56.3032, -5.6289) knots 0 0 0 0 0.269225 0.471143 0.471143 0.697796 1 1 1 1
  spline S119 degree 3 poles (-56.3032, -6.2037) (-56.2155, -6.2037) (-56.1214, -6.185) (-56.024, -6.0957) (-55.98, -6.0295) (-55.9693, -5.9515) (-55.9693, -5.9187) knots 0 0 0 0 0.533809 0.533809 0.800204 1 1 1 1
  line L43 (-57.9254, -6.2037) -> (-56.3032, -6.2037)
  spline S120 degree 3 poles (-58.3408, -5.7883) (-58.3408, -5.9007) (-58.3208, -6.0223) (-58.1617, -6.1836) (-58.0384, -6.2037) (-57.9254, -6.2037) knots 0 0 0 0 0.498542 0.498542 1 1 1 1
  line L44 (-58.3408, -3.5703) -> (-58.3408, -5.7883)
  spline S121 degree 3 poles (-57.9254, -3.1549) (-58.003, -3.1549) (-58.0826, -3.1644) (-58.1891, -3.2131) (-58.247, -3.2542) (-58.2849, -3.3126) (-58.3314, -3.4113) (-58.3408, -3.4918) (-58.3408, -3.5703) knots 0 0 0 0 0.345203 0.345203 0.519861 0.650854 0.650854 1 1 1 1
  line L45 (-56.3498, -3.1549) -> (-57.9254, -3.1549)
  spline S122 degree 3 poles (-56.0181, -3.4353) (-56.0181, -3.392) (-56.0323, -3.3151) (-56.0791, -3.2528) (-56.14, -3.1971) (-56.2239, -3.1612) (-56.3122, -3.1549) (-56.3498, -3.1549) knots 0 0 0 0 0.265144 0.464002 0.464002 0.770287 1 1 1 1
  spline S123 degree 3 poles (-56.3498, -3.7158) (-56.2623, -3.7158) (-56.1678, -3.6991) (-56.079, -3.6178) (-56.0322, -3.5556) (-56.0181, -3.4786) (-56.0181, -3.4353) knots 0 0 0 0 0.536345 0.536345 0.735054 1 1 1 1
  line L46 (-57.645, -3.7158) -> (-56.3498, -3.7158)
  line L47 (-57.645, -4.3396) -> (-57.645, -3.7158)
  line L48 (-56.4568, -4.3396) -> (-57.645, -4.3396)
  spline S124 degree 3 poles (-56.1345, -4.613) (-56.1345, -4.5708) (-56.1489, -4.496) (-56.1949, -4.4357) (-56.2451, -4.3898) (-56.322, -4.3484) (-56.4084, -4.3396) (-56.4568, -4.3396) knots 0 0 0 0 0.26597 0.465447 0.465447 0.694541 1 1 1 1
  spline S125 degree 3 poles (-56.4568, -4.8911) (-56.3709, -4.8911) (-56.2781, -4.8728) (-56.1858, -4.7838) (-56.1446, -4.7195) (-56.1345, -4.6446) (-56.1345, -4.613) knots 0 0 0 0 0.538356 0.538356 0.802153 1 1 1 1
  line L49 (-57.645, -4.8911) -> (-56.4568, -4.8911)
  line L50 (-57.645, -5.6289) -> (-57.645, -4.8911)
  spline S126 degree 3 poles (-56.0402, 13.0879) (-56.0758, 13.0879) (-56.1359, 13.0813) (-56.2125, 13.0458) (-56.2475, 13.0124) (-56.3076, 12.9323) (-56.3389, 12.8613) (-56.3621, 12.7889) knots 0 0 0 0 0.223548 0.37258 0.521612 0.521612 1 1 1 1
  spline S127 degree 3 poles (-55.7319, 12.7772) (-55.7319, 12.824) (-55.7478, 12.9063) (-55.7974, 12.9744) (-55.8551, 13.0312) (-55.9246, 13.0759) (-56.0059, 13.0879) (-56.0402, 13.0879) knots 0 0 0 0 0.288798 0.505397 0.505397 0.788027 1 1 1 1
  spline S128 degree 3 poles (-56.9875, 11.7451) (-56.7973, 11.7451) (-56.6043, 11.7731) (-56.2816, 11.911) (-56.1416, 12.0001) (-55.939, 12.2154) (-55.8571, 12.328) (-55.7612, 12.5557) (-55.7319, 12.6662) (-55.7319, 12.7772) knots 0 0 0 0 0.318995 0.318995 0.587325 0.587325 0.813706 0.813706 1 1 1 1
  spline S129 degree 3 poles (-58.0847, 12.1911) (-57.9997, 12.0909) (-57.8998, 12.0017) (-57.6732, 11.8664) (-57.5507, 11.8199) (-57.281, 11.7578) (-57.1328, 11.7451) (-56.9875, 11.7451) knots 0 0 0 0 0.323223 0.323223 0.642558 0.642558 1 1 1 1
  spline S130 degree 3 poles (-58.4595, 13.3172) (-58.4595, 13.1751) (-58.447, 13.0312) (-58.3903, 12.7609) (-58.3484, 12.6342) (-58.2351, 12.3981) (-58.166, 12.2887) (-58.0847, 12.1911) knots 0 0 0 0 0.35352 0.35352 0.683864 0.683864 1 1 1 1
  spline S131 degree 3 poles (-57.0038, 14.8963) (-57.1976, 14.8963) (-57.3954, 14.8605) (-57.7507, 14.7171) (-57.9137, 14.6076) (-58.1812, 14.3304) (-58.2852, 14.1561) (-58.4292, 13.7646) (-58.4595, 13.538) (-58.4595, 13.3172) knots 0 0 0 0 0.242459 0.242459 0.47899 0.47899 0.723758 0.723758 1 1 1 1
  spline S132 degree 3 poles (-55.7389, 13.9526) (-55.7389, 14.1059) (-55.8078, 14.2521) (-56.0098, 14.5378) (-56.1697, 14.6587) (-56.5459, 14.8515) (-56.7773, 14.8963) (-57.0038, 14.8963) knots 0 0 0 0 0.267231 0.267231 0.605244 0.605244 1 1 1 1
  spline S133 degree 3 poles (-56.0356, 13.6442) (-55.9904, 13.6442) (-55.911, 13.6622) (-55.8474, 13.7133) (-55.7939, 13.7711) (-55.751, 13.8394) (-55.7389, 13.919) (-55.7389, 13.9526) knots 0 0 0 0 0.287108 0.502439 0.502439 0.78676 1 1 1 1
  spline S134 degree 3 poles (-56.38, 13.9106) (-56.3585, 13.8698) (-56.3183, 13.7993) (-56.2684, 13.735) (-56.22, 13.6896) (-56.1534, 13.6523) (-56.0779, 13.6442) (-56.0356, 13.6442) knots 0 0 0 0 0.298168 0.521794 0.521794 0.72674 1 1 1 1
  spline S135 degree 3 poles (-56.9991, 14.3215) (-56.8732, 14.3215) (-56.7435, 14.2937) (-56.5259, 14.1449) (-56.4431, 14.0305) (-56.38, 13.9106) knots 0 0 0 0 0.481676 0.481676 1 1 1 1
  spline S136 degree 3 poles (-57.7544, 13.2962) (-57.7544, 13.5646) (-57.7129, 13.8486) (-57.4815, 14.144) (-57.3167, 14.2835) (-57.1033, 14.3215) (-56.9991, 14.3215) knots 0 0 0 0 0.562819 0.562819 0.78141 1 1 1 1
  spline S137 degree 3 poles (-57.02, 12.3199) (-57.1553, 12.3199) (-57.2923, 12.3514) (-57.524, 12.4993) (-57.608, 12.6163) (-57.7352, 12.9167) (-57.7544, 13.109) (-57.7544, 13.2962) knots 0 0 0 0 0.294428 0.294428 0.592546 0.592546 1 1 1 1
  spline S138 degree 3 poles (-56.3621, 12.7889) (-56.4124, 12.6527) (-56.4938, 12.524) (-56.7299, 12.3543) (-56.8772, 12.3199) (-57.02, 12.3199) knots 0 0 0 0 0.504048 0.504048 1 1 1 1
  line L51 (-55.8125, 30.4029) -> (-56.5824, 32.3058)
  spline S139 degree 3 poles (-55.7179, 30.0697) (-55.7179, 30.1029) (-55.7278, 30.1607) (-55.7598, 30.2721) (-55.7901, 30.3495) (-55.8125, 30.4029) knots 0 0 0 0 0.285973 0.500452 1 1 1 1
  spline S140 degree 3 poles (-56.0588, 29.7451) (-56.0078, 29.7451) (-55.9179, 29.7638) (-55.8443, 29.8187) (-55.7837, 29.8801) (-55.734, 29.9497) (-55.7179, 30.034) (-55.7179, 30.0697) knots 0 0 0 0 0.295724 0.517516 0.517516 0.793221 1 1 1 1
  spline S141 degree 3 poles (-56.4522, 30.1633) (-56.4305, 30.1091) (-56.4074, 30.0552) (-56.3744, 29.9804) (-56.3511, 29.9311) (-56.3236, 29.8833) (-56.2772, 29.824) (-56.2426, 29.796) (-56.1595, 29.7535) (-56.1084, 29.7451) (-56.0588, 29.7451) knots 0 0 0 0 0.28332 0.28332 0.397008 0.548591 0.548591 0.759302 0.759302 1 1 1 1
  line L52 (-56.5798, 30.5015) -> (-56.4522, 30.1633)
  line L53 (-57.7092, 30.5015) -> (-56.5798, 30.5015)
  line L54 (-57.839, 30.1547) -> (-57.7092, 30.5015)
  spline S142 degree 3 poles (-58.2163, 29.7451) (-58.1793, 29.7451) (-58.1166, 29.7518) (-58.0367, 29.7885) (-58.0002, 29.8232) (-57.9657, 29.8696) (-57.9334, 29.9269) (-57.8857, 30.0315) (-57.856, 30.1085) (-57.839, 30.1547) knots 0 0 0 0 0.184001 0.306669 0.429336 0.429336 0.592443 0.755551 1 1 1 1
  spline S143 degree 3 poles (-58.5526, 30.065) (-58.5526, 30.0171) (-58.5312, 29.9334) (-58.477, 29.8665) (-58.4155, 29.8074) (-58.341, 29.7588) (-58.2533, 29.7451) (-58.2163, 29.7451) knots 0 0 0 0 0.281581 0.492766 0.492766 0.782614 1 1 1 1
  spline S144 degree 3 poles (-58.4629, 30.3862) (-58.4873, 30.3263) (-58.5115, 30.2661) (-58.5445, 30.1594) (-58.5526, 30.112) (-58.5526, 30.065) knots 0 0 0 0 0.579167 0.579167 1 1 1 1
  line L55 (-57.7089, 32.3038) -> (-58.4629, 30.3862)
  spline S145 degree 3 poles (-57.1481, 32.8963) (-57.2272, 32.8963) (-57.3085, 32.8814) (-57.4377, 32.8078) (-57.4904, 32.7607) (-57.5719, 32.6402) (-57.6036, 32.5717) (-57.6567, 32.4354) (-57.6826, 32.3694) (-57.7089, 32.3038) knots 0 0 0 0 0.269082 0.269082 0.503026 0.503026 0.759618 0.759618 1 1 1 1
  spline S146 degree 3 poles (-56.5824, 32.3058) (-56.611, 32.3827) (-56.64, 32.46) (-56.6956, 32.5952) (-56.7258, 32.6515) (-56.8015, 32.7615) (-56.8541, 32.808) (-56.9843, 32.8821) (-57.0674, 32.8963) (-57.1481, 32.8963) knots 0 0 0 0 0.278017 0.278017 0.494933 0.494933 0.726733 0.726733 1 1 1 1
  spline S147 degree 3 poles (-41.3146, 38.5458) (-41.2688, 38.5458) (-41.1867, 38.5595) (-41.1216, 38.611) (-41.0471, 38.703) (-41.0131, 38.7815) (-40.9753, 38.8911) (-40.9608, 38.932) (-40.9431, 38.9759) (-40.9351, 38.9939) (-40.9308, 39.0028) (-40.9276, 39.0089) (-40.9256, 39.0123) (-40.9245, 39.0139) (-40.924, 39.0148) knots 0 0 0 0 0.208917 0.365604 0.365604 0.74824 0.74824 0.892103 0.946051 0.964034 0.982017 0.991009 0.995504 1 1 1 1
  spline S148 degree 3 poles (-41.5973, 38.8449) (-41.5973, 38.7997) (-41.5852, 38.7187) (-41.5403, 38.6508) (-41.4864, 38.5969) (-41.4215, 38.5561) (-41.3463, 38.5458) (-41.3146, 38.5458) knots 0 0 0 0 0.295249 0.516686 0.516686 0.792866 1 1 1 1
  spline S149 degree 3 poles (-40.5395, 39.7304) (-40.6971, 39.7304) (-40.857, 39.7097) (-41.1249, 39.6029) (-41.2407, 39.5343) (-41.4167, 39.36) (-41.4856, 39.2611) (-41.5712, 39.055) (-41.5973, 38.9501) (-41.5973, 38.8449) knots 0 0 0 0 0.309207 0.309207 0.564439 0.564439 0.793646 0.793646 1 1 1 1
  spline S150 degree 3 poles (-39.993, 39.6306) (-40.1636, 39.705) (-40.3534, 39.7304) (-40.5395, 39.7304) knots 0 0 0 0 1 1 1 1
  spline S151 degree 3 poles (-39.4911, 38.8402) (-39.4911, 38.9504) (-39.5129, 39.0625) (-39.5948, 39.2664) (-39.6552, 39.3619) (-39.8051, 39.5199) (-39.8951, 39.5849) (-39.993, 39.6306) knots 0 0 0 0 0.336501 0.336501 0.670162 0.670162 1 1 1 1
  spline S152 degree 3 poles (-40.7251, 37.2855) (-40.7248, 37.2858) (-40.7245, 37.2862) (-40.6741, 37.3482) (-40.6074, 37.4123) (-40.4707, 37.5372) (-40.389, 37.6057) (-40.2544, 37.7159) (-40.1094, 37.8356) (-39.964, 37.9574) (-39.8384, 38.0694) (-39.743, 38.1733) (-39.6634, 38.2913) (-39.5723, 38.4425) (-39.5086, 38.599) (-39.4911, 38.7687) (-39.4911, 38.8402) knots 0 0 0 0 0.000671 0.000671 0.117108 0.136514 0.272358 0.272358 0.390523 0.548077 0.548077 0.63684 0.755191 0.755191 0.895082 1 1 1 1
  spline S153 degree 3 poles (-40.7655, 37.2378) (-40.7529, 37.2538) (-40.7398, 37.2694) (-40.7257, 37.2848) (-40.7254, 37.2851) (-40.7251, 37.2855) knots 0 0 0 0 0.977173 0.977173 1 1 1 1
  line L56 (-39.8134, 37.2378) -> (-40.7655, 37.2378)
  spline S154 degree 3 poles (-39.4399, 36.9481) (-39.4399, 36.995) (-39.4575, 37.078) (-39.514, 37.1417) (-39.6173, 37.2217) (-39.7184, 37.2378) (-39.8134, 37.2378) knots 0 0 0 0 0.264865 0.463514 0.463514 1 1 1 1
  spline S155 degree 3 poles (-39.7552, 36.663) (-39.7065, 36.663) (-39.6202, 36.6737) (-39.5456, 36.7206) (-39.491, 36.7772) (-39.4505, 36.8416) (-39.4399, 36.9165) (-39.4399, 36.9481) knots 0 0 0 0 0.306499 0.536374 0.536374 0.801303 1 1 1 1
  line L57 (-41.2354, 36.663) -> (-39.7552, 36.663)
  spline S156 degree 3 poles (-41.6043, 36.9923) (-41.6043, 36.9433) (-41.5848, 36.8572) (-41.5318, 36.7874) (-41.4662, 36.7218) (-41.3769, 36.673) (-41.2774, 36.663) (-41.2354, 36.663) knots 0 0 0 0 0.266651 0.46664 0.46664 0.771417 1 1 1 1
  spline S157 degree 3 poles (-41.4183, 37.4084) (-41.4222, 37.4042) (-41.4299, 37.3957) (-41.4447, 37.3781) (-41.4657, 37.3506) (-41.5037, 37.2931) (-41.5299, 37.2415) (-41.5636, 37.1661) (-41.5906, 37.0973) (-41.6043, 37.0239) (-41.6043, 36.9923) knots 0 0 0 0 0.037271 0.074542 0.149084 0.260897 0.521795 0.521795 0.795055 1 1 1 1
  spline S158 degree 3 poles (-40.6191, 38.1506) (-40.6677, 38.1178) (-40.773, 38.0306) (-40.8753, 37.9386) (-41.1, 37.7321) (-41.2606, 37.5716) (-41.4183, 37.4084) knots 0 0 0 0 0.161027 0.376351 0.376351 1 1 1 1
  spline S159 degree 3 poles (-40.1427, 38.8286) (-40.1427, 38.7522) (-40.1633, 38.6759) (-40.2338, 38.5218) (-40.2896, 38.4452) (-40.4321, 38.2921) (-40.5239, 38.2177) (-40.6191, 38.1506) knots 0 0 0 0 0.267675 0.267675 0.592009 0.592009 1 1 1 1
  spline S160 degree 3 poles (-40.5512, 39.2231) (-40.4796, 39.2231) (-40.4078, 39.207) (-40.2838, 39.1409) (-40.2326, 39.092) (-40.1602, 38.9718) (-40.1427, 38.8996) (-40.1427, 38.8286) knots 0 0 0 0 0.339544 0.339544 0.662755 0.662755 1 1 1 1
  spline S161 degree 3 poles (-40.924, 39.0148) (-40.9124, 39.0325) (-40.8872, 39.067) (-40.8367, 39.1212) (-40.7334, 39.1994) (-40.6253, 39.2231) (-40.5512, 39.2231) knots 0 0 0 0 0.142857 0.285714 0.5 1 1 1 1
  spline S162 degree 3 poles (-21.9932, 39.8018) (-22.0342, 39.8018) (-22.1071, 39.7879) (-22.1677, 39.7466) (-22.2192, 39.6986) (-22.2808, 39.6299) (-22.3373, 39.5564) (-22.3685, 39.514) knots 0 0 0 0 0.249934 0.437385 0.437385 0.678638 1 1 1 1
  spline S163 degree 3 poles (-21.6384, 39.4027) (-21.6384, 39.4606) (-21.6483, 39.5771) (-21.7298, 39.7225) (-21.8623, 39.7928) (-21.9499, 39.8018) (-21.9932, 39.8018) knots 0 0 0 0 0.285714 0.571429 0.785714 1 1 1 1
  line L58 (-21.6384, 37.8957) -> (-21.6384, 39.4027)
  line L59 (-21.6022, 37.8957) -> (-21.6384, 37.8957)
  spline S164 degree 3 poles (-21.2101, 37.6176) (-21.2101, 37.6639) (-21.219, 37.7314) (-21.2698, 37.8109) (-21.3084, 37.8385) (-21.4166, 37.8872) (-21.511, 37.8957) (-21.6022, 37.8957) knots 0 0 0 0 0.251599 0.359427 0.503198 0.503198 1 1 1 1
  spline S165 degree 3 poles (-21.565, 37.3442) (-21.5141, 37.3442) (-21.4242, 37.3511) (-21.3399, 37.3847) (-21.2893, 37.4199) (-21.2555, 37.4522) (-21.2175, 37.5248) (-21.2101, 37.5832) (-21.2101, 37.6176) knots 0 0 0 0 0.300514 0.5259 0.5259 0.661357 0.796814 1 1 1 1
  line L60 (-21.6384, 37.3442) -> (-21.565, 37.3442)
  line L61 (-21.6384, 37.0195) -> (-21.6384, 37.3442)
  spline S166 degree 3 poles (-21.9397, 36.6646) (-21.8931, 36.6646) (-21.8107, 36.6798) (-21.7435, 36.7308) (-21.6931, 36.7863) (-21.6479, 36.8711) (-21.6384, 36.9662) (-21.6384, 37.0195) knots 0 0 0 0 0.266469 0.466321 0.466321 0.69504 1 1 1 1
  spline S167 degree 3 poles (-22.2411, 37.0195) (-22.2411, 36.927) (-22.2205, 36.8285) (-22.1273, 36.7243) (-22.0576, 36.6765) (-21.9746, 36.6646) (-21.9397, 36.6646) knots 0 0 0 0 0.531532 0.531532 0.799228 1 1 1 1
  line L62 (-22.2411, 37.3442) -> (-22.2411, 37.0195)
  line L63 (-23.2012, 37.3442) -> (-22.2411, 37.3442)
  spline S168 degree 3 poles (-23.6329, 37.7154) (-23.6329, 37.6578) (-23.6153, 37.5558) (-23.553, 37.4722) (-23.4848, 37.4106) (-23.3816, 37.3559) (-23.266, 37.3442) (-23.2012, 37.3442) knots 0 0 0 0 0.268776 0.470357 0.470357 0.697347 1 1 1 1
  spline S169 degree 3 poles (-23.4343, 38.0876) (-23.459, 38.0551) (-23.4837, 38.0226) (-23.53, 37.962) (-23.5503, 37.9328) (-23.5877, 37.8734) (-23.6041, 37.8429) (-23.6269, 37.7801) (-23.6329, 37.7475) (-23.6329, 37.7154) knots 0 0 0 0 0.285867 0.285867 0.533862 0.533862 0.775039 0.775039 1 1 1 1
  line L64 (-22.3685, 39.514) -> (-23.4343, 38.0876)
  line L65 (3.8414, 39.172) -> (4.8169, 39.172)
  spline S170 degree 3 poles (3.4562, 39.4757) (3.4562, 39.4255) (3.4711, 39.3359) (3.53, 39.2658) (3.6393, 39.1853) (3.7436, 39.172) (3.8414, 39.172) knots 0 0 0 0 0.270564 0.473487 0.473487 1 1 1 1
  spline S171 degree 3 poles (3.8414, 39.7445) (3.7894, 39.7445) (3.6975, 39.7393) (3.6092, 39.7155) (3.5507, 39.6885) (3.5137, 39.6618) (3.465, 39.5853) (3.4562, 39.5201) (3.4562, 39.4757) knots 0 0 0 0 0.289076 0.505882 0.505882 0.647059 0.752941 1 1 1 1
  line L66 (5.182, 39.7445) -> (3.8414, 39.7445)
  spline S172 degree 3 poles (5.5974, 39.4338) (5.5974, 39.486) (5.5832, 39.5793) (5.5221, 39.6523) (5.4526, 39.7011) (5.3506, 39.7378) (5.2427, 39.7445) (5.182, 39.7445) knots 0 0 0 0 0.263961 0.461931 0.461931 0.692532 1 1 1 1
  spline S173 degree 3 poles (4.7433, 37.8619) (4.8083, 38.0674) (4.8858, 38.2721) (5.0696, 38.6056) (5.1549, 38.7453) (5.3328, 38.9756) (5.4106, 39.0782) (5.5178, 39.2249) (5.5691, 39.3035) (5.5974, 39.394) (5.5974, 39.4338) knots 0 0 0 0 0.359695 0.359695 0.630423 0.630423 0.845071 0.845071 0.933602 1 1 1 1
  spline S174 degree 3 poles (4.5886, 37.0754) (4.6062, 37.1615) (4.6194, 37.2484) (4.6453, 37.4253) (4.6591, 37.5151) (4.6925, 37.6917) (4.7171, 37.7772) (4.7433, 37.8619) knots 0 0 0 0 0.328698 0.328698 0.668554 0.668554 1 1 1 1
  spline S175 degree 3 poles (4.2138, 36.6724) (4.2643, 36.6724) (4.3541, 36.6875) (4.4285, 36.7392) (4.5011, 36.8128) (4.5506, 36.9176) (4.5789, 37.028) (4.5886, 37.0754) knots 0 0 0 0 0.250824 0.438942 0.438942 0.759573 1 1 1 1
  spline S176 degree 3 poles (3.8938, 37.0599) (3.8938, 36.9594) (3.9135, 36.8531) (4.0118, 36.7376) (4.0865, 36.685) (4.1761, 36.6724) (4.2138, 36.6724) knots 0 0 0 0 0.533412 0.533412 0.800034 1 1 1 1